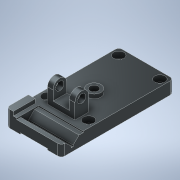
# Autodesk Inventor part: 4-上盖
Saved by Autodesk Inventor 2022 (Build 260153000, 153)
## iProperties
Created: 2023-01-07
Part Number: 4-上盖
Material: 灰口铁
Document SubType Name: Modeling
Designer: Lzy18
Density: 7.15 g/cm^3
Appearance: 灰口铁
Author: Lzy18
Autodesk Inventor part; units mm, degrees
ref_plane "XZ Plane" through (0, 0, 0) normal (0, 1, 0) x (-1, 0, 0)
ref_plane "XY Plane" through (0, 0, 0) normal (0, 0, 1) x (1, 0, 0)
sketch "草图1" plane through (0, 0, 0) normal (0, 1, 0) x (-1, 0, 0)
  line L0 (40, -82) -> (-40, -82)
  line L1 (-40, -82) -> (-40, 82)
  line L2 (-40, 82) -> (40, 82)
  line L3 (40, 82) -> (40, -82)
  line L4 (40, -82) -> (-40, 82) construction
  line L5 (-40, -82) -> (40, 82) construction
  point P0 (0, 0)
  dimension "d0" = 80
  dimension "d1" = 164
  constraints: 12 end point, 2 midpoint, 2 parallel, 1 horizontal, 1 perpendicular
  measures "d0" distance of L1.end L2.end
  measures "d1" distance of L0.end L1.end
extrude "拉伸1" add sketch "草图1" along normal blind 18
sketch "草图2" plane through (0, 18, 0) normal (0, 1, 0) x (1, 0, 0)
  line L0 (-40, -82) -> (40, -82) projected
  line L1 (-40, 82) -> (-40, -82) projected
  line L2 (-40, -82) -> (-40, -50)
  line L3 (-40, -50) -> (40, -50)
  line L4 (40, -50) -> (40, -82)
  line L5 (40, -82) -> (-40, -82)
  point P0 (0, 0)
  dimension "d4" = 32
  constraints: 8 end point, 2 parallel, 1 perpendicular, 1 point on line
  measures "d4" distance of L0.start L2.end
extrude "拉伸2" cut sketch "草图2" against normal blind 2
fillet "圆角1" radius 5 4 edges at (40, 8, 82) (40, 9, -82) (-40, 8, 82) (-40, 9, -82)
sketch "草图4" plane through (0, 0, 0) normal (1, 0, 0) x (0, 1, 0)
  line L0 (0, 82) -> (16, 82) projected
  line L1 (5.5, 66) -> (5.5, 64.5)
  line L2 (5.5, 64.5) -> (5.5, 67.5)
  line L3 (5.5, 64.5) -> (7.5, 64.5)
  line L4 (7.5, 67.5) -> (5.5, 67.5)
  line L5 (7.5, 64.5) -> (16, 56)
  line L6 (16, 77) -> (16, 50) projected
  line L7 (7.5, 67.5) -> (16, 76)
  line L8 (16, 76) -> (16, 56)
  line L9 (5.5, 66) -> (6, 66)
  point P0 (0, 0)
  dimension "d15" = 16
  dimension "d16" = 1.5
  dimension "d17" = 3
  dimension "d18" = 2
  constraints: 16 end point, 3 point on line, 1 collinear, 1 horizontal, 1 perpendicular, 1 vertical
  measures "d15" distance from line of L0 L1.start
  measures "d16" distance of L1.start L1.end
  measures "d17" distance of L1.end L2.end
  measures "d18" distance of L1.end L3.end
extrude "拉伸3" cut sketch "草图4" along normal blind 40 and the other way blind 25
sketch "草图6" plane through (0, 16, 0) normal (0, 1, 0) x (1, 0, 0)
  line L0 (40, -76) -> (-25, -76) projected
  line L1 (-25, -76) -> (-25, -56) projected
  line L2 (-25, -56) -> (40, -56) projected
  line L3 (40, -50) -> (40, -56) projected
  line L4 (-40, -50) -> (40, -50) projected
  line L5 (-40, -77) -> (-40, -50) projected
  arc A0 (-40, -77) -> (-35, -82) centre (-35, -77) ccw projected
  line L6 (35, -82) -> (-35, -82) projected
  arc A1 (35, -82) -> (40, -77) centre (35, -77) ccw projected
  line L7 (40, -76) -> (40, -77) projected
  line L8 (-40, -50) -> (40, -50) projected
  line L9 (-40, -50) -> (-30, -50)
  line L10 (-30, -50) -> (-30, -82)
  line L11 (-35, -82) -> (35, -82) projected
  point P0 (0, 0)
  dimension "d27" = 10
  constraints: 4 end point, 2 point on line, 1 perpendicular
  measures "d27" distance of L4.start L9.end
extrude "拉伸5" add sketch "草图6" along normal blind 8 contours L6 A0 L5 L4 L10
sketch "草图7" plane through (0, 16, 0) normal (0, 1, 0) x (1, 0, 0)
  line L0 (-30, -50) -> (-30, -82) projected
  line L1 (35, -82) -> (-30, -82) projected
  arc A0 (35, -82) -> (40, -77) centre (35, -77) ccw projected
  line L2 (40, -76) -> (40, -77) projected
  line L3 (40, -76) -> (-25, -76) projected
  line L4 (-25, -76) -> (-25, -56) projected
  line L5 (-25, -56) -> (40, -56) projected
  line L6 (40, -50) -> (40, -56) projected
  line L7 (-30, -50) -> (40, -50) projected
  line L8 (-30, -50) -> (40, -50) projected
  line L9 (-25, -50) -> (-25, -82)
  line L10 (35, -82) -> (-30, -82) projected
  point P0 (0, 0)
  constraints: 2 end point, 2 point on line, 1 perpendicular
extrude "拉伸6" add sketch "草图7" along normal blind 2 contours L7 L9 L4 L1 L0
sketch "草图8" plane through (0, 18, 0) normal (0, 1, 0) x (1, 0, 0)
  circle A0 centre (30, -32) radius 7.5
  line L0 (35, -82) -> (-25, -82) projected
  line L1 (40, -50) -> (40, 77) projected
  circle A1 centre (30, 72) radius 7.5
  line L2 (35, 82) -> (-35, 82) projected
  point P0 (0, 0)
  dimension "d32" = 15
  dimension "d34" = 10
  dimension "d35" = 15
  dimension "d36" = 10
  dimension "d38" = 50
  constraints: 2 centre point
  measures "d32" diameter of A0
  measures "d34" distance from line of L1 A0.centre
  measures "d35" diameter of A1
  measures "d36" distance from line of L2 A1.centre
  measures "d38" distance from line of L0 A0.centre
extrude "拉伸7" cut sketch "草图8" against normal blind 9
sketch "草图9" plane through (30, 9, -72) normal (0, 1, 0) x (1, 0, 0)
  circle A0 centre (0, 0) radius 7.5 projected
  circle A1 centre (0, -104) radius 7.5 projected
  point P0 (-30, -72)
  constraints: 2 coincident
hole "孔1" at (30, 9, -72) at (30, 9, 32) direction (0, -1, 0) diameter 10 end through all
mirror "镜像1" about plane through (0, 0, 0) normal (1, 0, 0) of "拉伸7", "孔1"
sketch "草图11" plane through (0, 18, 0) normal (0, 1, 0) x (1, 0, 0)
  circle A0 centre (0, 6) radius 10
  line L0 (35, -82) -> (-25, -82) projected
  point P0 (0, 0)
  dimension "d50" = 20
  dimension "d51" = 88
  constraints: 1 centre point
  measures "d50" diameter of A0
  measures "d51" distance from line of L0 A0.centre
extrude "拉伸8" add sketch "草图11" along normal blind 6
sketch "草图12" plane through (0, 24, -6) normal (0, 1, 0) x (1, 0, 0)
  circle A0 centre (0, 0) radius 6
  point P0 (0, -6)
  dimension "d54" = 12
  constraints: 1 centre point
  measures "d54" diameter of A0
extrude "拉伸9" cut sketch "草图12" against normal blind 15.5
sketch "草图13" plane through (0, 0, 0) normal (0, -1, 0) x (1, 0, 0)
  circle A0 centre (-30, -72) radius 5 projected
  circle A1 centre (-30, 32) radius 5 projected
  circle A2 centre (30, -72) radius 5 projected
  circle A3 centre (30, 32) radius 5 projected
  arc A4 (-40, -77) -> (-35, -82) centre (-35, -77) ccw projected
  line L0 (35, -82) -> (-35, -82) projected
  arc A5 (35, -82) -> (40, -77) centre (35, -77) ccw projected
  line L1 (40, 77) -> (40, -77) projected
  arc A6 (40, 77) -> (35, 82) centre (35, 77) ccw projected
  line L2 (-35, 82) -> (35, 82) projected
  arc A7 (-35, 82) -> (-40, 77) centre (-35, 77) ccw projected
  line L3 (-40, -77) -> (-40, 77) projected
  circle A8 centre (0, -6) radius 10
  point P0 (0, 0)
  dimension "d57" = 20
  dimension "d58" = 88
  constraints: 1 centre point
  measures "d57" diameter of A8
  measures "d58" distance from line of L2 A8.centre
extrude "拉伸10" cut sketch "草图13" against normal up to surface (8.5 mm away) contours A8
ref_plane "工作平面1" through (20, 0, 0) normal (1, 0, 0) x (0, 1, 0)
sketch "草图15" plane through (20, 0, 0) normal (1, 0, 0) x (0, 1, 0)
  line L0 (18, 4) -> (18, -16) projected
  line L1 (18, -64.5) -> (18, -79.5) projected
  line L2 (18, 39.5) -> (18, 24.5) projected
  line L3 (18, 39.5) -> (18, 24.5) projected
  line L4 (18, -64.5) -> (18, -79.5) projected
  line L5 (18, -77) -> (18, -82) projected
  line L6 (18, -77) -> (18, 50) projected
  line L7 (18, 82) -> (18, 50) projected
  line L8 (18, 82) -> (18, 50) projected
  line L9 (18, 50) -> (18, -77) projected
  line L10 (18, -82) -> (18, -77) projected
  line L11 (18, 39.5) -> (18, 24.5) projected
  line L12 (16, 82) -> (0, 82) projected
  line L13 (18, 50) -> (18, -77) projected
  line L14 (18, 42) -> (40, 42)
  line L15 (40, 22) -> (18, 22)
  line L16 (18, 22) -> (18, 42)
  arc A0 (40, 22) -> (40, 42) centre (40, 32) ccw
  point P0 (0, 0)
  point P1 (18, 32)
  dimension "d62" = 50
  dimension "d63" = 10
  dimension "d66" = 20
  dimension "d67" = 22
  constraints: 6 end point, 2 point on circle, 1 centre point, 1 horizontal, 1 midpoint, 1 parallel, 2 other
  measures "d62" distance from line of L12 point (18, 32)
  measures "d63" distance of point (18, 32) L14.start
  measures "d66" diameter of A0
  measures "d67" distance of point (18, 32) A0.centre
extrude "拉伸11" add sketch "草图15" against normal blind 8
sketch "草图16" plane through (12, 0, 0) normal (-1, 0, 0) x (0, 0, 1)
  line L0 (22, 40) -> (22, 18) projected
  line L1 (22, 18) -> (22, 40) projected
  line L2 (42, 18) -> (22, 18) projected
  line L3 (22, 26) -> (42, 26)
  line L4 (42, 26) -> (42, 18)
  line L5 (42, 18) -> (22, 18)
  line L6 (22, 18) -> (22, 26)
  point P0 (0, 0)
  dimension "d70" = 8
  constraints: 8 end point, 2 parallel, 1 horizontal, 1 perpendicular, 1 point on line
  measures "d70" distance from line of L2 L3.start
extrude "拉伸12" add sketch "草图16" along normal blind 12
sketch "草图17" plane through (20, 0, 0) normal (1, 0, 0) x (0, 0, -1)
  line L0 (-42, 40) -> (-42, 18) projected
  line L1 (-22, 18) -> (-42, 18) projected
  line L2 (-22, 18) -> (-22, 40) projected
  arc A0 (-22, 40) -> (-42, 40) centre (-32, 40) ccw projected
  circle A1 centre (-32, 40) radius 6
  point P0 (0, 0)
  dimension "d73" = 12
  constraints: 1 centre point, 1 coincident
  measures "d73" diameter of A1
extrude "拉伸13" cut sketch "草图17" against normal blind 8 contours A1
mirror "镜像2" about plane through (0, 0, 0) normal (1, 0, 0) of "拉伸11", "拉伸12", "拉伸13"
sketch "草图18" plane through (0, 0, 0) normal (0, -1, 0) x (1, 0, 0)
  line L0 (12, 22) -> (12, 42) projected
  circle A0 centre (0, -6) radius 10 projected
  circle A1 centre (-30, -72) radius 5 projected
  circle A2 centre (-30, 32) radius 5 projected
  circle A3 centre (30, -72) radius 5 projected
  circle A4 centre (30, 32) radius 5 projected
  arc A5 (-40, -77) -> (-35, -82) centre (-35, -77) ccw projected
  line L1 (35, -82) -> (-35, -82) projected
  arc A6 (35, -82) -> (40, -77) centre (35, -77) ccw projected
  line L2 (40, 77) -> (40, -77) projected
  arc A7 (40, 77) -> (35, 82) centre (35, 77) ccw projected
  line L3 (-35, 82) -> (35, 82) projected
  arc A8 (-35, 82) -> (-40, 77) centre (-35, 77) ccw projected
  line L4 (-40, -77) -> (-40, 77) projected
  line L5 (-35, 82) -> (35, 82) projected
  line L6 (35, -82) -> (-35, -82) projected
  line L7 (20, 82) -> (-20, 82)
  line L8 (-20, 82) -> (-20, -82)
  line L9 (-20, -82) -> (20, -82)
  line L10 (20, -82) -> (20, 82)
  point P0 (0, 0)
  dimension "d76" = 20
  dimension "d77" = 40
  constraints: 8 end point, 2 parallel, 2 point on line, 1 horizontal, 1 perpendicular
  measures "d76" horizontal distance of A0.centre L7.start
  measures "d77" distance of L9.end L8.end
extrude "拉伸14" cut sketch "草图18" against normal blind 2 contours L8 L3 L10 L1
